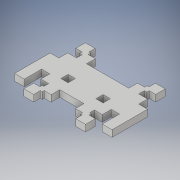
# Autodesk Inventor part: Monster3
Saved by Autodesk Inventor 2019 (Build 230136000, 136)
## iProperties
Created: 2018-12-04
Part Number: Monster3
Material: Generic
Document SubType Name: Modeling
Designer: Administrator
Density: 1 g/cm^3
Appearance: Default
Author: Administrator
Autodesk Inventor part; units mm, degrees
ref_plane "YZ Plane" through (0, 0, 0) normal (1, 0, 0) x (0, 1, 0)
ref_plane "XZ Plane" through (0, 0, 0) normal (0, 1, 0) x (-1, 0, 0)
ref_plane "XY Plane" through (0, 0, 0) normal (0, 0, 1) x (1, 0, 0)
sketch "Sketch1" plane through (0, 0, 0) normal (0, 1, 0) x (-1, 0, 0)
  line L0 (0, 0) -> (441.3397, 0) construction
  line L1 (441.3397, 0) -> (441.3397, -197.552) construction
  line L2 (441.3397, -197.552) -> (0, -197.552) construction
  line L3 (0, -197.552) -> (0, 0) construction
  line L4 (171.126, -125.5766) -> (171.126, -117.3504)
  line L5 (171.126, -117.3504) -> (164.413, -117.3504)
  line L6 (164.413, -117.3504) -> (164.413, -115.3958)
  line L7 (164.413, -115.3958) -> (162.5492, -115.3958)
  line L8 (162.5492, -115.3958) -> (162.5492, -109.1021)
  line L9 (162.5492, -109.1021) -> (153.1492, -109.1021)
  line L10 (153.1492, -109.1021) -> (153.1492, -118.4751)
  line L11 (153.1492, -118.4751) -> (159.1458, -118.4751)
  line L12 (159.1458, -118.4751) -> (159.1458, -120.6901)
  line L13 (159.1458, -120.6901) -> (160.7124, -120.6901)
  line L14 (160.7124, -120.6901) -> (160.7124, -125.2266)
  line L15 (160.7124, -125.2266) -> (153.1492, -125.2266)
  line L16 (153.1492, -125.2266) -> (153.1492, -133.9258)
  line L17 (153.1492, -133.9258) -> (145.278, -133.9258)
  line L18 (145.278, -133.9258) -> (145.278, -117.3504)
  line L19 (145.278, -117.3504) -> (135.8674, -117.3504)
  line L20 (135.8674, -117.3504) -> (135.8674, -151.5449)
  line L21 (135.8674, -151.5449) -> (144.3246, -151.5449)
  line L22 (144.3246, -151.5449) -> (144.3246, -160.0944)
  line L23 (144.3246, -160.0944) -> (152.8126, -160.0944)
  line L24 (152.8126, -160.0944) -> (152.8126, -165.4456)
  line L25 (152.8126, -165.4456) -> (150.4138, -165.4456)
  line L26 (150.4138, -165.4456) -> (150.4138, -167.7828)
  line L27 (150.4138, -167.7828) -> (144.3246, -167.7828)
  line L28 (144.3246, -167.7828) -> (144.3246, -177.0397)
  line L29 (144.3246, -177.0397) -> (153.766, -177.0397)
  line L30 (153.766, -177.0397) -> (153.766, -170.9505)
  line L31 (153.766, -170.9505) -> (155.5804, -170.9505)
  line L32 (155.5804, -170.9505) -> (155.5804, -168.5671)
  line L33 (155.5804, -168.5671) -> (162.4692, -168.5671)
  line L34 (162.4692, -168.5671) -> (162.4692, -160.0944)
  line L35 (162.4692, -135.3817) -> (169.4041, -135.3817)
  line L36 (169.4041, -135.3817) -> (169.4041, -142.3165)
  line L37 (169.4041, -142.3165) -> (162.4692, -142.3165)
  line L38 (162.4692, -142.3165) -> (162.4692, -135.3817)
  line L39 (162.4692, -160.0944) -> (182.7899, -160.0944)
  line L40 (171.126, -125.5766) -> (182.7899, -125.5766)
  line L41 (194.4538, -125.5766) -> (194.4538, -117.3504)
  line L42 (194.4538, -117.3504) -> (201.1668, -117.3504)
  line L43 (201.1668, -117.3504) -> (201.1668, -115.3958)
  line L44 (201.1668, -115.3958) -> (203.0306, -115.3958)
  line L45 (203.0306, -115.3958) -> (203.0306, -109.1021)
  line L46 (203.0306, -109.1021) -> (212.4307, -109.1021)
  line L47 (212.4307, -109.1021) -> (212.4307, -118.4751)
  line L48 (212.4307, -118.4751) -> (206.4341, -118.4751)
  line L49 (206.4341, -118.4751) -> (206.4341, -120.6901)
  line L50 (206.4341, -120.6901) -> (204.8674, -120.6901)
  line L51 (204.8674, -120.6901) -> (204.8674, -125.2266)
  line L52 (204.8674, -125.2266) -> (212.4307, -125.2266)
  line L53 (212.4307, -125.2266) -> (212.4307, -133.9258)
  line L54 (212.4307, -133.9258) -> (220.3018, -133.9258)
  line L55 (220.3018, -133.9258) -> (220.3018, -117.3504)
  line L56 (220.3018, -117.3504) -> (229.7124, -117.3504)
  line L57 (229.7124, -117.3504) -> (229.7124, -151.5449)
  line L58 (229.7124, -151.5449) -> (221.2552, -151.5449)
  line L59 (221.2552, -151.5449) -> (221.2552, -160.0944)
  line L60 (221.2552, -160.0944) -> (212.7672, -160.0944)
  line L61 (212.7672, -160.0944) -> (212.7672, -165.4456)
  line L62 (212.7672, -165.4456) -> (215.166, -165.4456)
  line L63 (215.166, -165.4456) -> (215.166, -167.7828)
  line L64 (215.166, -167.7828) -> (221.2552, -167.7828)
  line L65 (221.2552, -167.7828) -> (221.2552, -177.0397)
  line L66 (221.2552, -177.0397) -> (211.8138, -177.0397)
  line L67 (211.8138, -177.0397) -> (211.8138, -170.9505)
  line L68 (211.8138, -170.9505) -> (209.9994, -170.9505)
  line L69 (209.9994, -170.9505) -> (209.9994, -168.5671)
  line L70 (209.9994, -168.5671) -> (203.1106, -168.5671)
  line L71 (203.1106, -168.5671) -> (203.1106, -160.0944)
  line L72 (203.1106, -135.3817) -> (196.1757, -135.3817)
  line L73 (196.1757, -135.3817) -> (196.1757, -142.3165)
  line L74 (196.1757, -142.3165) -> (203.1106, -142.3165)
  line L75 (203.1106, -142.3165) -> (203.1106, -135.3817)
  line L76 (203.1106, -160.0944) -> (182.7899, -160.0944)
  line L77 (194.4538, -125.5766) -> (182.7899, -125.5766)
  dimension "d17" = 90
  dimension "d18" = 6.9349
  dimension "d21" = 6.9349
  dimension "d22" = 26.6019
  constraints: 148 end point, 27 perpendicular, 8 point on line, 4 horizontal, 2 parallel, 1 vertical, 2 other
  measures "d17" angle of L15 L16
  measures "d18" distance of L37.end L35.start
  measures "d21" distance of L35.start L35.end
  measures "d22" distance between parallel lines of L20 L38
extrude "Extrusion1" add sketch "Sketch1" along normal blind 6.35
equation "\"d21\" = d18"
body "Solid1"
